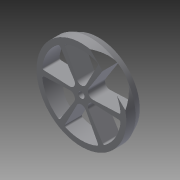
# Autodesk Inventor part: Colossus_7kW_Rotor
Saved by Autodesk Inventor 2014 (Build 180170000, 170)
## iProperties
Created: 2014-11-23
Part Number: Colossus_7kW_Rotor
Material: Générique
Document SubType Name: Modeling
Designer: Yann
Density: 1 g/cm^3
Appearance: Par défaut
Author: Yann
Autodesk Inventor part; units mm, degrees
ref_plane "YZ Plane" through (0, 0, 0) normal (1, 0, 0) x (0, 1, 0)
ref_plane "XZ Plane" through (0, 0, 0) normal (0, 1, 0) x (-1, 0, 0)
ref_plane "XY Plane" through (0, 0, 0) normal (0, 0, 1) x (1, 0, 0)
sketch "Esquisse1" plane through (0, 0, 0) normal (0, 1, 0) x (-1, 0, 0)
  arc A0 (29.4095, 49.2352) -> (-29.4095, 49.2352) centre (0, 0) ccw
  circle A1 centre (0, 0) radius 57.35
  line L0 (0, -80.29) -> (0, 80.29) construction
  line L1 (-80.29, 0) -> (80.29, 0) construction
  circle A2 centre (0, 0) radius 4
  line L2 (-5.7656, 13.9986) -> (-21.0747, 43.4072)
  line L3 (21.0747, 43.4072) -> (5.7656, 13.9986)
  arc A3 (20.099, 46.1644) -> (-20.099, 46.1644) centre (0, 0) ccw
  arc A4 (-5.7656, 13.9986) -> (5.7656, 13.9986) centre (0, 17) ccw
  arc A5 (-20.099, 46.1644) -> (-21.0747, 43.4072) centre (-19.3007, 44.3307) ccw
  arc A6 (21.0747, 43.4072) -> (20.099, 46.1644) centre (19.3007, 44.3307) ccw
  line L4 (-15.006, 2.0062) -> (-48.129, 3.4524)
  line L5 (-27.0544, 39.9548) -> (-9.2404, 11.9924)
  arc A7 (-29.93, 40.4885) -> (-50.0291, 5.6759) centre (0, 0) ccw
  arc A8 (-15.006, 2.0062) -> (-9.2404, 11.9924) centre (-14.7224, 8.5) ccw
  arc A9 (-50.0291, 5.6759) -> (-48.129, 3.4524) centre (-48.0418, 5.4505) ccw
  arc A10 (-27.0544, 39.9548) -> (-29.93, 40.4885) centre (-28.7411, 38.8802) ccw
  line L6 (-9.2404, -11.9924) -> (-27.0544, -39.9548)
  line L7 (-48.129, -3.4524) -> (-15.006, -2.0062)
  arc A11 (-50.0291, -5.6759) -> (-29.93, -40.4885) centre (0, 0) ccw
  arc A12 (-9.2404, -11.9924) -> (-15.006, -2.0062) centre (-14.7224, -8.5) ccw
  arc A13 (-29.93, -40.4885) -> (-27.0544, -39.9548) centre (-28.7411, -38.8802) ccw
  arc A14 (-48.129, -3.4524) -> (-50.0291, -5.6759) centre (-48.0418, -5.4505) ccw
  line L8 (5.7656, -13.9986) -> (21.0747, -43.4072)
  line L9 (-21.0747, -43.4072) -> (-5.7656, -13.9986)
  arc A15 (-20.099, -46.1644) -> (20.099, -46.1644) centre (0, 0) ccw
  arc A16 (5.7656, -13.9986) -> (-5.7656, -13.9986) centre (0, -17) ccw
  arc A17 (20.099, -46.1644) -> (21.0747, -43.4072) centre (19.3007, -44.3307) ccw
  arc A18 (-21.0747, -43.4072) -> (-20.099, -46.1644) centre (-19.3007, -44.3307) ccw
  line L10 (15.006, -2.0062) -> (48.129, -3.4524)
  line L11 (27.0544, -39.9548) -> (9.2404, -11.9924)
  arc A19 (29.93, -40.4885) -> (50.0291, -5.6759) centre (0, 0) ccw
  arc A20 (15.006, -2.0062) -> (9.2404, -11.9924) centre (14.7224, -8.5) ccw
  arc A21 (50.0291, -5.6759) -> (48.129, -3.4524) centre (48.0418, -5.4505) ccw
  arc A22 (27.0544, -39.9548) -> (29.93, -40.4885) centre (28.7411, -38.8802) ccw
  line L12 (9.2404, 11.9924) -> (27.0544, 39.9548)
  line L13 (48.129, 3.4524) -> (15.006, 2.0062)
  arc A23 (50.0291, 5.6759) -> (29.93, 40.4885) centre (0, 0) ccw
  arc A24 (9.2404, 11.9924) -> (15.006, 2.0062) centre (14.7224, 8.5) ccw
  arc A25 (29.93, 40.4885) -> (27.0544, 39.9548) centre (28.7411, 38.8802) ccw
  arc A26 (48.129, 3.4524) -> (50.0291, 5.6759) centre (48.0418, 5.4505) ccw
  circle A27 centre (0, 0) radius 16 construction
  circle A28 centre (0, 0) radius 57.35 construction
  point P0 (0, 2.9231)
  point P1 (-22.0435, 45.2682)
  point P2 (22.0435, 45.2682)
  point P3 (-2.5315, 1.4615)
  point P4 (-50.2251, 3.5439)
  point P5 (-28.1817, 41.7243)
  point P6 (-2.5315, -1.4615)
  point P7 (-28.1817, -41.7243)
  point P8 (-50.2251, -3.5439)
  point P9 (0, -2.9231)
  point P10 (22.0435, -45.2682)
  point P11 (-22.0435, -45.2682)
  point P12 (2.5315, -1.4615)
  point P13 (50.2251, -3.5439)
  point P14 (28.1817, -41.7243)
  point P15 (2.5315, 1.4615)
  point P16 (28.1817, 41.7243)
  point P17 (50.2251, 3.5439)
  dimension "d0" = 8
  dimension "d1" = 6.5
  dimension "d2" = 2
  dimension "d3" = 7
  dimension "d4" = 17
  dimension "d5" = 55
  dimension "d8" = 360
  constraints: 62 point on circle, 27 centre point, 25 point on line, 24 end point, 7 tangent, 3 coincident, 2 equal radius, 1 symmetric about line, 115 other
  measures "d0" diameter of A2
  measures "d1" radius of A4
  measures "d2" radius of A5
  measures "d3" radial gap between concentric circles of A3 A1
  measures "d4" distance of A4.centre A2.centre
  measures "d5" angle of L3 L2
extrude "Extrusion1" add sketch "Esquisse1" against normal blind 22
chamfer "Chanfrein1" distance 10 angle 25 1 edges at (57.35, 0, 0) measured on face at (57.35, -0.5, 0)
